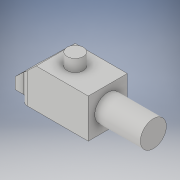
# Autodesk Inventor part: 18 pin schieter
Saved by Autodesk Inventor 2019 (Build 230136000, 136)
## iProperties
Created: 2021-01-19
Part Number: 18 pin schieter
Material: Generic
Document SubType Name: Modeling
Designer: Stefan
Density: 1 g/cm^3
Appearance: Default
Author: Stefan
Autodesk Inventor part; units mm, degrees
ref_plane "YZ Plane" through (0, 0, 0) normal (1, 0, 0) x (0, 1, 0)
ref_plane "XZ Plane" through (0, 0, 0) normal (0, 1, 0) x (-1, 0, 0)
ref_plane "XY Plane" through (0, 0, 0) normal (0, 0, 1) x (1, 0, 0)
sketch "Sketch1" plane through (0, 0, 0) normal (1, 0, 0) x (0, 1, 0)
  line L0 (-6, 6) -> (6, 6)
  line L1 (6, 6) -> (6, -6)
  line L2 (6, -6) -> (-6, -6)
  line L3 (-6, -6) -> (-6, 6)
  line L4 (-6, 6) -> (6, -6) construction
  line L5 (6, 6) -> (-6, -6) construction
  point P0 (0, 0)
  dimension "d0" = 12
  dimension "d1" = 12
  constraints: 12 end point, 2 midpoint, 2 parallel, 1 horizontal, 1 perpendicular
  measures "d0" distance of L1.end L2.end
  measures "d1" distance of L0.end L1.end
extrude "Extrusion1" add sketch "Sketch1" along normal blind 20
sketch "Sketch2" plane through (0, -6, 6) normal (0, 0, 1) x (1, 0, 0)
  line L0 (0, 0) -> (0, 12) projected
  line L1 (0, 12) -> (-6.9282, 0)
  line L2 (0, 12) -> (15.674, 12) construction
  line L3 (0, 0) -> (-6.9282, 0)
  line L4 (0, 0) -> (20, 0) projected
  line L5 (0, 0) -> (0, 12)
  point P0 (0, 6)
  dimension "d4" = 120
  constraints: 8 end point, 2 horizontal, 1 perpendicular
  measures "d4" angle of L1 L2
extrude "Extrusion2" add sketch "Sketch2" against normal blind 12
sketch "Sketch3" plane through (20, 0, 0) normal (1, 0, 0) x (0, 0, -1)
  circle A0 centre (0, 0) radius 4
  dimension "d7" = 8
  constraints: 1 centre point, 1 coincident
  measures "d7" diameter of A0
extrude "Extrusion3" add sketch "Sketch3" along normal blind 14
sketch "Sketch4" plane through (20, 6, 6) normal (0, 1, 0) x (1, 0, 0)
  circle A0 centre (-10, 6) radius 2.5
  line L0 (-20, 0) -> (-20, 12) projected
  line L1 (-20, 0) -> (0, 0) projected
  point P0 (-20, 6)
  dimension "d10" = 5
  dimension "d11" = 10
  dimension "d12" = 6
  constraints: 1 centre point
  measures "d10" diameter of A0
  measures "d11" distance from line of A0.centre L0
  measures "d12" distance from line of L1 A0.centre
extrude "Extrusion4" add sketch "Sketch4" along normal blind 3.75
sketch "Sketch5" plane through (20, -6, 6) normal (0, 0, 1) x (1, 0, 0)
  line L0 (0, 0) -> (-26.9282, 0) projected
  line L1 (-26.9282, 0) -> (-24.9282, 0)
  line L2 (-24.9282, 0) -> (-24.9282, 3.4641)
  line L3 (-26.9282, 0) -> (-20, 12) projected
  line L4 (-26.9282, 0) -> (-24.9282, 3.4641)
  point P0 (-20, 6)
  dimension "d15" = 2
  constraints: 6 end point, 2 point on line, 1 perpendicular
  measures "d15" distance of L0.end L1.end
extrude "Extrusion5" cut sketch "Sketch5" against normal blind 12
sketch "Sketch6" plane through (-4.9282, -6, 6) normal (-1, 0, 0) x (0, 0, 1)
  line L0 (0, 0) -> (-12, 0) projected
  line L1 (0, 0) -> (-2.5, 0)
  line L2 (-2.5, 0) -> (-2.5, 12)
  line L3 (-12, 12) -> (0, 12) projected
  line L4 (-2.5, 12) -> (0, 12)
  line L5 (0, 12) -> (0, 0)
  line L6 (-12, 0) -> (-12, 3.4641) projected
  line L7 (-12, 0) -> (-9.5, 0)
  line L8 (-9.5, 0) -> (-9.5, 12)
  line L9 (-9.5, 12) -> (-12, 12)
  line L10 (-12, 3.4641) -> (-12, 12) projected
  line L11 (-12, 12) -> (-12, 0)
  point P0 (-6, 6)
  dimension "d18" = 2.5
  dimension "d19" = 2.5
  constraints: 16 end point, 4 point on line, 3 collinear, 2 perpendicular, 1 vertical
  measures "d18" distance of L0.start L1.end
  measures "d19" distance of L0.end L7.end
extrude "Extrusion6" cut sketch "Sketch6" against normal blind 4.5 contours L0 L2 L3 L5 | L0 L6 L10 L3 L8
fillet "Fillet1" radius 2 4 edges at (-0.4282, -0.3708, 3.5) (-0.4282, -0.3708, -3.5) (-0.4282, -0.3708, -6) (-0.4282, -0.3708, 6)
sketch "Sketch7" plane through (20, -6, 6) normal (0, 0, 1) x (1, 0, 0)
  line L0 (-20, 12) -> (-18.7201, 12) projected
  line L1 (-20, 12) -> (-16, 12)
  line L2 (-20.5742, 11.0055) -> (-22.4282, 7.7942) projected
  line L3 (-16, 12) -> (-22.4282, 7.7942)
  line L4 (-22.4282, 7.7942) -> (-20, 12)
  point P0 (-20, 6)
  dimension "d23" = 4
  constraints: 6 end point, 2 collinear
  measures "d23" distance of L0.start L1.end
extrude "Extrusion7" cut sketch "Sketch7" against normal blind 20
sketch "Sketch8" plane through (20, -6, 6) normal (0, 0, 1) x (1, 0, 0)
  line L0 (-16, 12) -> (-18.7201, 10.2203) projected
  line L1 (-24.9282, 3.4641) -> (-22.4282, 7.7942) projected
  line L2 (-16, 12) -> (-24.9282, 3.4641)
  line L3 (-24.9282, 3.4641) -> (-24.9282, 12)
  line L4 (-16, 12) -> (0, 12) projected
  line L5 (-24.9282, 12) -> (-16, 12)
  point P0 (-20, 6)
  constraints: 6 end point, 1 perpendicular, 1 vertical
extrude "Extrusion8" cut sketch "Sketch8" against normal blind 20
body "Solid1"
